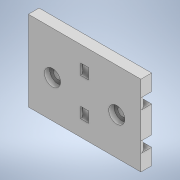
# Autodesk Inventor part: ESC_Halter
Saved by Autodesk Inventor 2021 (Build 250183000, 183)
## iProperties
Created: 2024-05-18
Part Number: ESC_Halter
Material: Generic
Document SubType Name: Modeling
Designer: Lukas
Density: 1 g/cm^3
Appearance: Default
Author: Lukas
Autodesk Inventor part; units mm, degrees
ref_plane "YZ Plane" through (0, 0, 0) normal (1, 0, 0) x (0, 1, 0)
ref_plane "XZ Plane" through (0, 0, 0) normal (0, 1, 0) x (-1, 0, 0)
ref_plane "XY Plane" through (0, 0, 0) normal (0, 0, 1) x (1, 0, 0)
sketch "Sketch1" plane through (0, 0, 0) normal (0, 0, 1) x (1, 0, 0)
  line L0 (-21, 15) -> (21, 15)
  line L1 (21, 15) -> (21, -15)
  line L2 (21, -15) -> (-21, -15)
  line L3 (-21, -15) -> (-21, 15)
  circle A0 centre (-12, -1) radius 1.6
  circle A1 centre (12, -1) radius 1.6
  line L4 (-1.5, -5) -> (1.5, -5)
  line L5 (1.5, -5) -> (1.5, -9)
  line L6 (1.5, -9) -> (-1.5, -9)
  line L7 (-1.5, -9) -> (-1.5, -5)
  line L8 (-1.5, 9) -> (1.5, 9)
  line L9 (1.5, 9) -> (1.5, 5)
  line L10 (1.5, 5) -> (-1.5, 5)
  line L11 (-1.5, 5) -> (-1.5, 9)
  point P0 (0, 0)
  point P1 (-21, 0)
  point P2 (0, 15)
  point P3 (0, 5)
  point P4 (0, -5)
  dimension "d0" = 30
  dimension "d1" = 42
  dimension "d2" = 24
  dimension "d3" = 12
  dimension "d4" = 14
  dimension "d5" = 3.2
  dimension "d8" = 6
  dimension "d9" = 6
  dimension "d10" = 4
  dimension "d11" = 3
  constraints: 24 end point, 6 parallel, 4 midpoint, 3 horizontal, 3 perpendicular, 3 vertical alignment, 2 centre point, 2 equal length, 2 horizontal alignment, 1 equal radius
  measures "d0" distance of L0.end L1.end
  measures "d1" distance of L0.start L0.end
  measures "d2" distance of A1.centre A0.centre
  measures "d3" horizontal distance of point (0, 0) A0.centre
  measures "d4" distance from line of L2 A0.centre
  measures "d5" diameter of A0
  measures "d8" distance between parallel lines of L0 L8
  measures "d9" distance between parallel lines of L2 L6
  measures "d10" distance of L8.end L9.end
  measures "d11" distance of L8.start L8.end
extrude "Extrusion1" add sketch "Sketch1" along normal blind 4
sketch "Sketch2" plane through (0, 0, 0) normal (0, 0, -1) x (-1, 0, 0)
  line L0 (1.5, -5) -> (-1.5, -5) projected
  line L1 (21, 15) -> (21, -15) projected
  line L2 (1.5, -5) -> (21, -5)
  line L3 (21, -5) -> (21, -9)
  line L4 (21, -9) -> (1.5, -9)
  line L5 (1.5, -9) -> (1.5, -5)
  line L6 (-21, -15) -> (-21, 15) projected
  line L7 (-1.5, -5) -> (-21, -5)
  line L8 (-21, -5) -> (-21, -9)
  line L9 (-21, -9) -> (-1.5, -9)
  line L10 (-1.5, -9) -> (-1.5, -5)
  line L11 (-1.5, 9) -> (-1.5, 5) projected
  line L12 (-1.5, 5) -> (-21, 5)
  line L13 (-21, 5) -> (-21, 9)
  line L14 (-21, 9) -> (-1.5, 9)
  line L15 (-1.5, 9) -> (-1.5, 5)
  line L16 (1.5, 5) -> (1.5, 9) projected
  line L17 (21, 15) -> (21, -15) projected
  line L18 (1.5, 5) -> (21, 5)
  line L19 (21, 5) -> (21, 9)
  line L20 (21, 9) -> (1.5, 9)
  line L21 (1.5, 9) -> (1.5, 5)
  point P0 (0, 0)
  point P1 (21, 9)
  point P2 (21, 5)
  point P3 (-21, 9)
  constraints: 32 end point, 8 parallel, 4 horizontal, 4 perpendicular, 4 point on line
extrude "Extrusion2" cut sketch "Sketch2" against normal blind 2
fillet "Fillet1" radius 2 8 edges at (21, 7, 2) (21, -7, 2) (1.5, -7, 2) (-1.5, -7, 2) (1.5, 7, 2) (-1.5, 7, 2) (-21, 7, 2) (-21, -7, 2)
sketch "Sketch3" plane through (0, 0, 4) normal (0, 0, 1) x (1, 0, 0)
  circle A0 centre (-12, -1) radius 1.6 projected
  circle A1 centre (-12, -1) radius 1.6 projected
  circle A2 centre (12, -1) radius 1.6 projected
  circle A3 centre (12, -1) radius 1.6 projected
  circle A4 centre (-12, -1) radius 1.6 projected
  circle A5 centre (-12, -1) radius 3
  circle A6 centre (12, -1) radius 3
  point P0 (0, 0)
  dimension "d15" = 6
  constraints: 2 centre point, 2 coincident, 1 equal radius
  measures "d15" diameter of A5
extrude "Extrusion3" cut sketch "Sketch3" against normal blind 2
equation "\"d3\" = 0.5 * d2"
equation "\"d9\" = d8"
body "Solid1"
